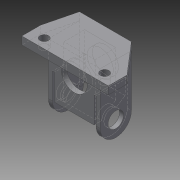
# Autodesk Inventor part: chain_end_extruder
Saved by Autodesk Inventor 2014 (Build 180170000, 170)
## iProperties
Created: 2016-05-16
Part Number: chain_end_extruder
Material: Generic
Document SubType Name: Modeling
Designer: 101767
Density: 1 g/cm^3
Appearance: Default
Author: 101767
Autodesk Inventor part; units mm, degrees
ref_plane "YZ Plane" through (0, 0, 0) normal (1, 0, 0) x (0, 1, 0)
ref_plane "XZ Plane" through (0, 0, 0) normal (0, 1, 0) x (-1, 0, 0)
sketch "Sketch1" plane through (0, 0, 0) normal (0, 0, 1) x (1, 0, 0)
  line L0 (0, 0) -> (15.2, 0)
  line L1 (15.2, 0) -> (15.2, 12)
  line L2 (15.2, 12) -> (0, 12)
  line L3 (0, 12) -> (0, 0)
  line L4 (1.6, 10) -> (13.6, 10)
  line L5 (13.6, 10) -> (13.6, 2)
  line L6 (13.6, 2) -> (1.6, 2)
  line L7 (1.6, 2) -> (1.6, 10)
  dimension "d0" = 15.2
  dimension "d1" = 12
  dimension "d2" = 1.6
  dimension "d3" = 2
  dimension "d4" = 2
  dimension "d5" = 1.6
  constraints: 16 end point, 4 parallel, 2 horizontal, 2 perpendicular
  measures "d0" distance of L1.end L2.end
  measures "d1" distance of L0.end L1.end
  measures "d2" distance between parallel lines of L3 L7
  measures "d3" distance between parallel lines of L2 L4
  measures "d4" distance between parallel lines of L0 L6
  measures "d5" distance between parallel lines of L1 L5
extrude "Extrusion1" add sketch "Sketch1" along normal blind 20
sketch "Sketch2" plane through (0, 0, 0) normal (1, 0, 0) x (0, 1, 0)
  line L0 (0, 0) -> (12, 0) construction
  line L1 (6, 13.0663) -> (6, -2.0093) construction
  line L2 (0, 0) -> (0, 20) construction
  line L3 (12, 0) -> (12, 20) construction
  line L4 (6, 0) -> (12, 3.8224)
  line L5 (12, 3.8224) -> (12, 0)
  line L6 (12, 0) -> (6, 0)
  dimension "d8" = 12
  dimension "d9" = 6
  dimension "d10" = 32.5
  constraints: 8 end point, 2 collinear, 2 point on line, 1 midpoint, 1 perpendicular
  measures "d8" distance of L0.start L0.end
  measures "d9" distance between parallel lines of L2 L1
  measures "d10" angle of L0 L4
extrude "Extrusion2" cut sketch "Sketch2" along normal through all
sketch "Sketch9" plane through (0, 0, 20) normal (-1, 0, 0) x (0, 0, 1)
  line L0 (-20, 0) -> (0, 0) construction
  line L1 (0, 12) -> (0, 0) construction
  line L2 (-16.1776, 12) -> (0, 12) construction
  line L3 (-20, 0) -> (-20, 14.5103) construction
  line L4 (-20, 0) -> (0, 0)
  line L5 (0, 12) -> (0, 0)
  line L6 (0, 12) -> (-20, 12)
  arc A0 (-20, 12) -> (-20, 0) centre (-20, 6) ccw
  constraints: 8 end point, 4 perpendicular, 2 point on circle, 2 tangent, 1 centre point, 1 point on line
extrude "Extrusion8" add sketch "Sketch9" along normal blind 2.4
sketch "Sketch4" plane through (1.6, 2, 20) normal (1, 0, 0) x (0, 0, -1)
  circle A0 centre (20, 4) radius 3
  point P0 (20, -2)
  dimension "d14" = 6
  constraints: 1 centre point, 1 coincident
  measures "d14" diameter of A0
extrude "Extrusion3" cut sketch "Sketch4" along normal through all both and the other way through all
sketch "Sketch11" plane through (15.2, 12, 20) normal (0, 1, 0) x (1, 0, 0)
  line L0 (0, 0) -> (-17.6, 0) construction
  line L1 (-15.2, 26) -> (-15.2, 20) construction
  line L2 (-15.2, 26) -> (-16, 26)
  line L3 (-16, 26) -> (-16, 10)
  line L4 (-16, 10) -> (-15.2, 10)
  line L5 (-15.2, 10) -> (-15.2, 26)
  line L6 (-15.2, 20) -> (-13.6, 20) construction
  dimension "d38" = 10
  dimension "d39" = 0.8
  constraints: 8 end point, 2 parallel, 1 horizontal, 1 perpendicular
  measures "d38" distance between parallel lines of L4 L6
  measures "d39" distance of L3.end L4.end
extrude "Extrusion9" cut sketch "Sketch11" against normal through all
ref_plane "Work Plane4" through (7.6, 2, 20) normal (-1, 0, 0) x (0, 0, 1)
mirror "Mirror3" about plane through (7.6, 2, 20) normal (-1, 0, 0) of "Extrusion8", "Extrusion3", "Extrusion9"
sketch "Sketch14" plane through (0, 0, 20) normal (0, 0, 1) x (1, 0, 0)
  line L0 (17.6, 0) -> (-2.4, 0) construction
  line L1 (-2.4, 12) -> (17.6, 12) construction
  line L2 (-5.4, 0) -> (-5.4, -7.2)
  line L3 (-5.4, -7.2) -> (27.9, -7.2)
  line L4 (27.9, -7.2) -> (27.9, 0)
  line L5 (17.6, 12) -> (-2.4, 12)
  line L6 (-5.4, -3.6) -> (27.9, -3.6) construction
  circle A0 centre (-0.4, -3.6) radius 1.65
  line L7 (7.6, 12) -> (7.6, -12.1697) construction
  circle A1 centre (22.9, -3.6) radius 1.65
  line L8 (-5.4, 0) -> (-2.4, 12)
  line L9 (17.6, 12) -> (27.9, 0)
  point P0 (0, 0)
  dimension "d54" = 7.2
  dimension "d55" = 3.3
  dimension "d56" = 8
  dimension "d57" = 15.3
  dimension "d58" = 5
  dimension "d59" = 5
  constraints: 16 end point, 4 parallel, 3 midpoint, 3 point on line, 2 centre point, 1 collinear, 1 equal radius, 1 perpendicular
  measures "d54" distance of L2.start L2.end
  measures "d55" diameter of A0
  measures "d56" distance from line of A0.centre L7
  measures "d57" distance from line of L7 A1.centre
  measures "d58" distance from line of L2 A0.centre
  measures "d59" distance from line of A1.centre L4
extrude "Extrusion12" add sketch "Sketch14" along normal blind 3
sketch "Sketch15" plane through (-2.4, 0, 0) normal (0, -1, 0) x (1, 0, 0)
  line L0 (2.4, 0) -> (17.6, 0) construction
  line L1 (17.6, 10) -> (18.4, 10) construction
  line L2 (10, 0) -> (10, 23.7385) construction
  circle A0 centre (10, 12) radius 5
  dimension "d62" = 10
  dimension "d63" = 12
  constraints: 2 end point, 1 centre point, 1 midpoint, 1 perpendicular, 1 point on line
  measures "d62" diameter of A0
  measures "d63" distance from line of L0 A0.centre
extrude "Extrusion13" cut sketch "Sketch15" against normal through all
equation "\"d9\" = 0.5 * d8"
body "Solid1"
